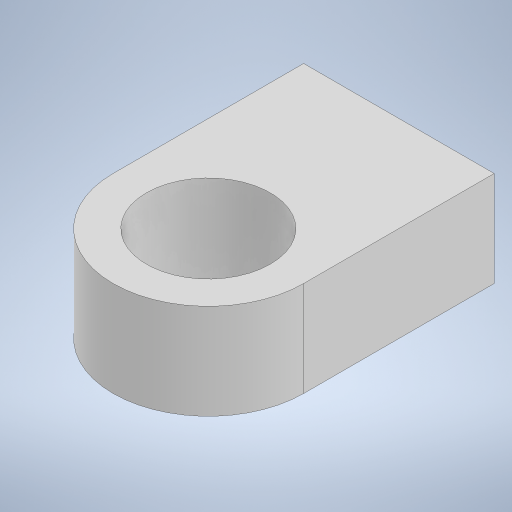
# Autodesk Inventor part: 05-17-2023 cardine superiore analisi fem
Saved by Autodesk Inventor 2023 (Build 270158000, 158)
## iProperties
Created: 2023-05-17
Part Number: 05-17-2023 cardine superiore analisi fem
Material: Generico
Document SubType Name: Modeling
Designer: Admin
Density: 1 g/cm^3
Appearance: Default
Author: Admin
Autodesk Inventor part; units mm, degrees
ref_plane "YZ Plane" through (0, 0, 0) normal (1, 0, 0) x (0, 1, 0)
ref_plane "XZ Plane" through (0, 0, 0) normal (0, 1, 0) x (-1, 0, 0)
ref_plane "XY Plane" through (0, 0, 0) normal (0, 0, 1) x (1, 0, 0)
sketch "Schizzo2" plane through (0, 0, 0) normal (0, 1, 0) x (-1, 0, 0)
  circle A0 centre (0, 0) radius 6.5
  circle A1 centre (0, 0) radius 10
  line L0 (10, 0) -> (10, -20)
  line L1 (10, -20) -> (-10, -20)
  line L2 (-10, -20) -> (-10, 0)
  line L3 (0, 0) -> (0, -33.9201) construction
  line L4 (0, 0) -> (14.6717, 0) construction
  dimension "d0" = 13
  dimension "d1" = 20
  dimension "d2" = 20
  constraints: 10 end point, 2 centre point, 2 coincident, 2 point on circle, 2 tangent, 1 horizontal, 1 parallel, 1 perpendicular, 1 vertical, 1 other
  measures "d0" diameter of A0
  measures "d1" diameter of A1
  measures "d2" distance of L0.start L0.end
extrude "Estrusione1" add sketch "Schizzo2" along normal blind 10
